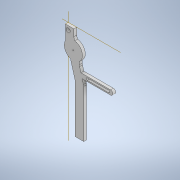
# Autodesk Inventor part: P5
Saved by Autodesk Inventor 2022 (Build 260153000, 153)
## iProperties
Created: 2022-11-21
Part Number: P5
Material: Genérico
Document SubType Name: Modeling
Designer: javie
Density: 1 g/cm^3
Appearance: Valor por defecto
Author: javie
Autodesk Inventor part; units mm, degrees
ref_plane "YZ Plane" through (0, 0, 0) normal (1, 0, 0) x (0, 1, 0)
ref_plane "XZ Plane" through (0, 0, 0) normal (0, 1, 0) x (-1, 0, 0)
ref_plane "XY Plane" through (0, 0, 0) normal (0, 0, 1) x (1, 0, 0)
sketch "Boceto1" plane through (0, 0, 0) normal (0, 0, 1) x (1, 0, 0)
  circle A0 centre (5, -7) radius 3.5
  line L0 (38.7297, -66.7617) -> (75.9094, -66.7617)
  arc A1 (75.9094, -66.7617) -> (75.9094, -62.7617) centre (75.9094, -64.7617) ccw
  line L1 (75.9094, -62.7617) -> (38.7297, -62.7617)
  arc A2 (38.7297, -62.7617) -> (38.7297, -66.7617) centre (38.7297, -64.7617) ccw
  arc A3 (0, -25.4308) -> (9.3356, -48.4983) centre (13.9922, -33.1909) ccw
  line L2 (0, -25.4308) -> (0, 0)
  line L3 (0, 0) -> (14.9941, 0)
  line L4 (14.9941, 0) -> (14.9941, -11.843)
  arc A4 (14.9941, -11.843) -> (16.6942, -17.4207) centre (24.9941, -11.843) ccw
  line L5 (24.7137, -45.0673) -> (24.7137, -49.8402)
  arc A5 (24.7137, -49.8402) -> (25.0885, -52.5523) centre (34.7137, -49.8402) ccw
  line L6 (25.0885, -52.5523) -> (27.4017, -60.7617)
  line L7 (27.4017, -60.7617) -> (79.4017, -60.7617)
  arc A6 (79.4017, -68.7617) -> (79.4017, -60.7617) centre (79.6579, -64.7617) ccw
  line L8 (79.4017, -68.7617) -> (29.656, -68.7617)
  line L9 (29.656, -68.7617) -> (31.8389, -76.5087)
  arc A7 (32.2137, -79.2209) -> (31.8389, -76.5087) centre (22.2137, -79.2209) ccw
  line L10 (32.2137, -79.2209) -> (32.2137, -163.1909)
  line L11 (32.2137, -163.1909) -> (17.2137, -163.1909)
  line L12 (17.2137, -163.1909) -> (17.2137, -79.2209)
  arc A8 (17.2137, -79.2209) -> (16.8389, -76.5087) centre (7.2137, -79.2209) ccw
  line L13 (16.8389, -76.5087) -> (10.0234, -52.321)
  arc A9 (9.6811, -50.4155) -> (10.0234, -52.321) centre (19.6486, -49.6089) ccw
  arc A10 (9.6811, -50.4155) -> (9.3356, -48.4983) centre (-0.2863, -51.2221) ccw
  arc A11 (24.7137, -45.0673) -> (16.6942, -17.4207) centre (13.9922, -33.1909) ccw
  circle A12 centre (13.9922, -33.1909) radius 1
  point P0 (38.7297, -66.7617)
  point P1 (0, -25.4308)
  point P2 (9.3356, -48.4983)
  point P3 (9.6811, -50.4155)
  point P4 (31.8389, -76.5087)
  point P5 (25.0885, -52.5523)
  point P6 (16.6942, -17.4207)
  dimension "d0" = 2
  constraints: 28 end point, 22 point on circle, 13 centre point, 1 coincident
  measures "d0" diameter of A12
extrude "Extrusión1" add sketch "Boceto1" along normal blind 5
